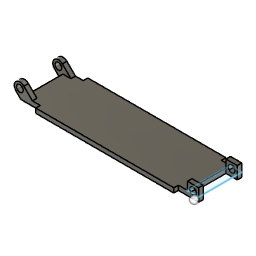
電源蓋 v3 (Autodesk Fusion 360 design; units mm, degrees)
Autodesk Fusion 360 part; units mm, degrees
sketch "スケッチ1" plane through (0, 0, 0) normal (0, 0, 1) x (1, 0, 0)
  line L0 (0, 0) -> (77, 0)
  line L1 (77, 0) -> (77, -23)
  line L2 (77, -23) -> (0, -23)
  line L3 (0, -23) -> (0, 0)
  dimension "d1" = 77
  dimension "d2" = 23
  constraint horizontal L0
  constraint vertical L1
  constraint horizontal L2
  constraint vertical L3
  constraint coincident L0.start L3.end
  measures "d1" distance of L0.start L0.end
  measures "d2" distance of L0.start L2.end
extrude "押し出し1" add sketch "スケッチ1" along normal blind 2
sketch "スケッチ2" plane through (0, 0, 0) normal (0, 0, 1) x (1, 0, 0)
sketch "スケッチ3" plane through (0, 0, 0) normal (0, 1, 0) x (1, 0, 0)
  line L0 (77, 0) -> (77, -5.5)
  line L1 (77, 0) -> (72, 0)
  line L2 (72, 0) -> (72, -5.5)
  line L3 (72, -5.5) -> (77, -5.5)
  circle A0 centre (74.5, -3) radius 1.5
  line L4 (77, -2) -> (75.618, -2)
  line L5 (73.382, -2) -> (72, -2)
  arc A1 (75.618, -2) -> (73.382, -2) centre (74.5, -3) ccw
  dimension "d5" = 5.5
  dimension "d6" = 5.5
  dimension "d8" = 3
  constraint vertical L0
  constraint perpendicular L0 L1
  constraint perpendicular L1 L2
  constraint coincident L0 L4.start
  constraint coincident A0 L4.end
  constraint perpendicular L0 L4
  constraint coincident A0 L5.start
  constraint coincident L2 L5.end
  constraint perpendicular L2 L5
  constraint coincident A0.centre A1.centre
  measures "d5" distance of L0.start L0.end
  measures "d6" distance of L1.end L2.end
  measures "d8" diameter of A0
extrude "押し出し2" add sketch "スケッチ3" against normal blind 23 contours L0 L2 L3 A0 L4 L5
sketch "スケッチ4" plane through (0, 0, 0) normal (0, 1, 0) x (1, 0, 0)
  circle A0 centre (74.5, -3) radius 1.5
extrude "押し出し3" cut sketch "スケッチ4" against normal blind 23
sketch "スケッチ5" plane through (0, 0, 0) normal (0, 0, 1) x (1, 0, 0)
  line L0 (77, -23) -> (77, -21)
  line L1 (77, -21) -> (72, -21)
  line L2 (72, -21) -> (72, -2)
  line L3 (72, -2) -> (77, -2)
  line L4 (77, -2) -> (77, -21)
  constraint vertical L0
  constraint horizontal L1
  constraint vertical L2
  constraint horizontal L3
  constraint vertical L4
sketch "スケッチ6" plane through (0, 0, 0) normal (0, 1, 0) x (1, 0, 0)
sketch "スケッチ7" plane through (0, 0, 0) normal (0, 0, 1) x (1, 0, 0)
  line L0 (77, 0) -> (72, 0)
  line L1 (72, 0) -> (72, -2)
  line L2 (72, -2) -> (77, -2)
  line L3 (77, -2) -> (77, 0)
  line L4 (77, -21) -> (72, -21)
  line L5 (72, -21) -> (72, -23)
  line L6 (72, -23) -> (77, -23)
  line L7 (77, -23) -> (77, -21)
  constraint horizontal L0
  constraint vertical L1
  constraint horizontal L2
  constraint vertical L3
  constraint horizontal L4
  constraint vertical L5
  constraint horizontal L6
  constraint vertical L7
extrude "押し出し4" cut sketch "スケッチ7" along normal blind 10
sketch "スケッチ8" plane through (0, 0, 0) normal (0, 0, 1) x (1, 0, 0)
  line L0 (77, -2) -> (77, -4)
  line L1 (72, -21) -> (72, -19)
  line L2 (77, -4) -> (72, -4)
  line L3 (72, -4) -> (72, -19)
  line L4 (72, -19) -> (77, -19)
  line L5 (77, -19) -> (77, -4)
  constraint vertical L0
  constraint vertical L1
  constraint horizontal L2
  constraint vertical L3
  constraint horizontal L4
  constraint vertical L5
extrude "押し出し5" cut sketch "スケッチ8" along normal blind 20
sketch "スケッチ9" plane through (0, 0, 0) normal (0, 1, 0) x (1, 0, 0)
  circle A0 centre (-2, -4) radius 1.5
  arc A1 (-3.7678, -2.2322) -> (-0.2322, -5.7678) centre (-2, -4) ccw
  line L0 (-2, -4) -> (-3.7678, -2.2322) construction
  line L1 (-2, -4) -> (-0.2322, -5.7678) construction
  line L2 (0, -2) -> (7.5, -2)
  line L3 (-0.2322, -5.7678) -> (3.5355, -2)
  line L4 (-3.7678, -2.2322) -> (-1.5586, -0.023)
  line L5 (-1.5586, -0.023) -> (0, 0)
  line L6 (0, 0) -> (0, -2)
  dimension "d17" = 3
  dimension "d18" = 2.5
  dimension "d19" = 180
  constraint coincident A0.centre A1.centre
  constraint horizontal L2
  constraint coincident L2 L3.end
  constraint tangent A1 L3
  constraint tangent A1 L4
  constraint coincident L5.end L6.start
  constraint perpendicular L2 L6
  measures "d17" diameter of A0
  measures "d18" radius of A1
  measures "d19" angle of L0 L1
extrude "押し出し6" add sketch "スケッチ9" against normal blind 23
sketch "スケッチ10" plane through (0, 0, 0) normal (0, 0, 1) x (1, 0, 0)
  line L0 (0, 0) -> (0, -2)
  line L1 (0, -20) -> (0, -21)
  line L2 (0, -21) -> (-5, -21)
  line L3 (-5, -21) -> (0, -21)
  line L4 (0, -21) -> (0, -23)
  line L5 (0, -23) -> (-5, -23)
  line L6 (-5, -23) -> (-5, -21)
  line L7 (0, 0) -> (-5, 0)
  line L8 (-5, 0) -> (-5, -2)
  line L9 (-5, -2) -> (0, -2)
  line L10 (0, -2) -> (0, 0)
  constraint coincident L0.start L7.start
  constraint vertical L0
  constraint vertical L1
  constraint perpendicular L1 L2
  constraint horizontal L3
  constraint vertical L4
  constraint horizontal L5
  constraint vertical L6
  constraint horizontal L7
  constraint vertical L8
  constraint horizontal L9
  constraint vertical L10
extrude "押し出し7" cut sketch "スケッチ10" along normal blind 30
sketch "スケッチ11" plane through (0, 0, 0) normal (0, 0, 1) x (1, 0, 0)
  line L0 (0, -2) -> (0, -4)
  line L1 (0, -18) -> (0, -19)
  line L2 (0, -19) -> (-6, -19)
  line L3 (-6, -19) -> (0, -19)
  line L4 (0, -19) -> (0, -4)
  line L5 (0, -4) -> (-6, -4)
  line L6 (-6, -4) -> (-6, -19)
  constraint vertical L0
  constraint vertical L1
  constraint perpendicular L1 L2
  constraint horizontal L3
  constraint vertical L4
  constraint horizontal L5
  constraint vertical L6
extrude "押し出し8" cut sketch "スケッチ11" along normal blind 30
move_body "移動1" bodies 1 to x (1, 0, 0) y (0, 1, 0) z (0, 0, 1) at (0, 0, -2)
sketch "スケッチ12" plane through (0, 0, 0) normal (0, 0, 1) x (1, 0, 0)
  line L0 (0, -21) -> (3.5382, -21)
  line L1 (3.5382, -21) -> (3.5382, -23.0866)
  line L2 (3.5382, -23.0866) -> (0, -23.0866)
  line L3 (0, -23.0866) -> (0, -21)
  line L4 (0, -2) -> (3.5382, -2)
  line L5 (3.5382, -2) -> (3.5382, 0.1058)
  line L6 (3.5382, 0.1058) -> (0, 0.1058)
  line L7 (0, 0.1058) -> (0, -2)
  line L8 (0, -4) -> (5, -4)
  line L9 (5, -4) -> (5, -19)
  line L10 (5, -19) -> (0, -19)
  line L11 (0, -19) -> (0, -4)
  constraint horizontal L0
  constraint vertical L1
  constraint horizontal L2
  constraint vertical L3
  constraint horizontal L4
  constraint vertical L5
  constraint horizontal L6
  constraint vertical L7
  constraint horizontal L8
  constraint vertical L9
  constraint horizontal L10
  constraint vertical L11
extrude "押し出し9" cut sketch "スケッチ12" along normal blind 20 contours L8 L9 L10 L11
sketch "スケッチ13" plane through (0, 0, 0) normal (0, 0, 1) x (1, 0, 0)
  line L0 (0, 0) -> (5, 0)
  line L1 (5, 0) -> (5, -2)
  line L2 (5, -2) -> (0, -2)
  line L3 (0, -2) -> (0, 0)
  line L4 (0, -23) -> (5, -23)
  line L5 (5, -23) -> (5, -21)
  line L6 (5, -21) -> (0, -21)
  line L7 (0, -21) -> (0, -23)
  constraint horizontal L0
  constraint vertical L1
  constraint horizontal L2
  constraint vertical L3
  constraint coincident L0.start L3.end
  constraint horizontal L4
  constraint vertical L5
  constraint horizontal L6
  constraint vertical L7
extrude "押し出し10" cut sketch "スケッチ13" along normal blind 90
sketch "スケッチ14" plane through (0, 0, 0) normal (0, 0, 1) x (1, 0, 0)
  line L0 (0, 0) -> (7, 0)
  line L1 (7, 0) -> (7, -2)
  line L2 (7, -2) -> (0, -2)
  line L3 (0, -2) -> (0, 0)
  line L4 (0, -23) -> (7, -23)
  line L5 (7, -23) -> (7, -21)
  line L6 (7, -21) -> (0, -21)
  line L7 (0, -21) -> (0, -23)
  constraint horizontal L0
  constraint vertical L1
  constraint horizontal L2
  constraint vertical L3
  constraint coincident L0.start L3.end
  constraint horizontal L4
  constraint vertical L5
  constraint horizontal L6
  constraint vertical L7
extrude "押し出し11" cut sketch "スケッチ14" against normal blind 3
sketch "スケッチ15" plane through (0, 0, 0) normal (0, 0, 1) x (1, 0, 0)
  line L0 (72, 0) -> (68, 0)
  line L1 (68, 0) -> (68, -2)
  line L2 (68, -2) -> (72, -2)
  line L3 (72, -2) -> (72, 0)
  line L4 (72, -23) -> (68, -23)
  line L5 (68, -23) -> (68, -21)
  line L6 (68, -21) -> (72, -21)
  line L7 (72, -21) -> (72, -23)
  constraint horizontal L0
  constraint vertical L1
  constraint horizontal L2
  constraint vertical L3
  constraint horizontal L4
  constraint vertical L5
  constraint horizontal L6
  constraint vertical L7
extrude "押し出し12" cut sketch "スケッチ15" against normal blind 3
sketch "スケッチ16" plane through (0, 0, 0) normal (0, 1, 0) x (1, 0, 0)
